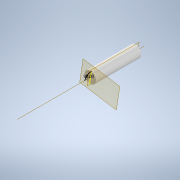
# Autodesk Inventor part: handle piston 2
Saved by Autodesk Inventor 2021 (Build 250183000, 183)
## iProperties
Created: 2021-03-12
Part Number: handle piston 2
Material: Generic
Document SubType Name: Modeling
Designer: ben
Density: 1 g/cm^3
Appearance: Default
Author: ben
Autodesk Inventor part; units mm, degrees
ref_plane "YZ Plane" through (0, 0, 0) normal (1, 0, 0) x (0, 1, 0)
ref_plane "XZ Plane" through (0, 0, 0) normal (0, 1, 0) x (-1, 0, 0)
ref_plane "XY Plane" through (0, 0, 0) normal (0, 0, 1) x (1, 0, 0)
sketch "Sketch1" plane through (0, 0, 0) normal (0, 0, 1) x (1, 0, 0)
  circle A0 centre (0, 0) radius 4.995
  dimension "d0" = 9.99
  constraints: 1 centre point, 1 coincident
  measures "d0" diameter of A0
ref_plane "Work Plane1" through (-67.8691, -14.8785, 98.7425) normal (-0.6355519, 0.0961754, -0.7660444) x (0.1496223, 0.9887432, 0)
ref_plane "Work Plane2" through (0, 0, 36.9492) normal (0, 0, 1) x (0.9887432, -0.1496223, 0)
ref_plane "Work Plane3" through (4.9388, -0.7474, 40.1113) normal (0, 0, 1) x (0.9887432, -0.1496223, 0)
extrude "Extrusion2" add sketch "Sketch1" along normal up to surface (40.1113 mm away)
ref_plane "Work Plane6" through (0, 0, 0) normal (0.9887432, -0.1496223, 0) x (0, 0, 1)
ref_plane "Work Plane5" through (-34.239, 15.2951, 36.9492) normal (-0.1496223, -0.9887432, 0) x (0.9887432, -0.1496223, 0)
sketch "Sketch4" plane through (0, 0, 0) normal (0.9887432, -0.1496223, 0) x (0, 0, 1)
  line L0 (40.1113, 4.995) -> (40.1113, -4.995) projected
  arc A0 (40.1113, -4.995) -> (45.1063, 0) centre (40.1113, 0) ccw
  line L1 (40.1113, 0) -> (45.1063, 0) construction
  line L2 (40.1113, 0) -> (40.1113, -4.995) construction
  line L3 (45.1063, 0) -> (40.1113, 0)
  line L4 (-9.2282, 0) -> (55.3689, 0) projected
  point P0 (0, 0)
  dimension "d6" = 90
  constraints: 6 end point, 2 point on circle, 1 centre point, 1 collinear, 1 midpoint
  measures "d6" angle of L2 L1
revolve "Revolution1" add sketch "Sketch4" angle 360 about axis through (0, 0, 0) along (0, 0, 1)
body "Solid1"
